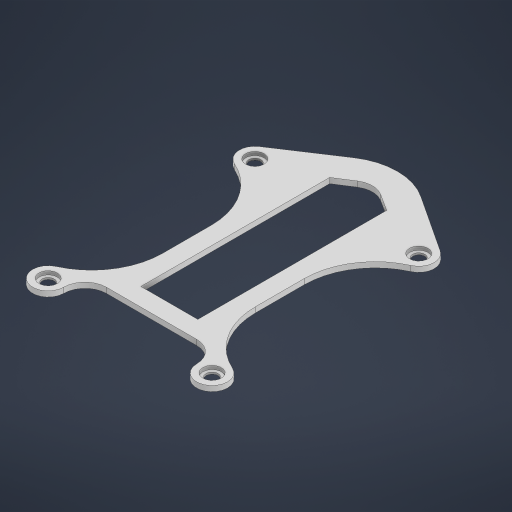
# Autodesk Inventor part: Skirt
Saved by Autodesk Inventor 2023 (Build 270158000, 158)
## iProperties
Created: 2022-10-14
Part Number: Skirt
Material: 一般
Document SubType Name: Modeling
Designer: hide
Density: 1 g/cm^3
Appearance: 既定
Author: hide
Autodesk Inventor part; units mm, degrees
ref_plane "YZ Plane" through (0, 0, 0) normal (1, 0, 0) x (0, 1, 0)
ref_plane "XZ Plane" through (0, 0, 0) normal (0, 1, 0) x (-1, 0, 0)
ref_plane "XY Plane" through (0, 0, 0) normal (0, 0, 1) x (1, 0, 0)
sketch "スケッチ1" plane through (0, 0, 0) normal (0, 1, 0) x (-1, 0, 0)
  circle A0 centre (11.5, 0) radius 0.85
  circle A1 centre (11.5, 29) radius 0.85
  line L0 (0, -11.6446) -> (0, 36.0381)
  arc A2 (12.3932, 27.0169) -> (9.325, 29) centre (11.5, 29) ccw
  arc A3 (12.6962, -1.8165) -> (12.3932, 1.9831) centre (11.5, 0) ccw
  circle A4 centre (0, 0) radius 5
  line L1 (4, 23.5) -> (4, -3)
  line L2 (4, -3) -> (1.6185, -4.5259)
  line L3 (12.6962, -1.8165) -> (4.675, -7.0989)
  arc A5 (0, -8.5) -> (4.675, -7.0989) centre (0, 0) ccw
  circle A6 centre (0, -2) radius 3
  line L4 (4, 23.5) -> (0, 23.5)
  line L5 (14.3325, 28.15) -> (9.1092, 28.15)
  line L6 (-4, 23.5) -> (-4, -3)
  line L7 (-4, -3) -> (-1.6185, -4.5259)
  line L8 (-4, 23.5) -> (0, 23.5)
  line L9 (6.5, 11.1009) -> (6.5, 17.8991)
  arc A7 (6.325, 26) -> (9.325, 29) centre (6.325, 29) ccw
  line L10 (6.325, 26) -> (0, 26)
  arc A8 (12.3932, 27.0169) -> (6.5, 17.8991) centre (16.5, 17.8991) ccw
  arc A9 (6.5, 11.1009) -> (12.3932, 1.9831) centre (16.5, 11.1009) ccw
  circle A10 centre (11.5, 0) radius 1.175
  circle A11 centre (11.5, 29) radius 1.175
  point P0 (0, 30.9357)
  point P1 (4, 3)
  point P2 (0, 26.5)
  point P3 (0, -5)
  point P4 (-1.6185, -4.5259)
  point P5 (0, 1)
  point P6 (-4, 3)
  point P7 (0, -5)
  point P8 (3.4728, -6.6475)
  point P9 (0, 5)
  point P10 (0, -5)
  point P11 (2.7322, -4.1875)
  point P12 (-4, -3)
  dimension "d7" = 10
  dimension "d2" = 29
  dimension "d18" = 8.5
  dimension "d24" = 1.7
  dimension "d25" = 2
  dimension "d39" = 8
  dimension "d41" = 2.5
  dimension "d43" = 2.5
  dimension "d44" = 10
  dimension "d45" = 23
  dimension "d47" = 3
  dimension "d48" = 2.35
  dimension "d49" = 1
  dimension "d50" = 1
  constraints: 20 end point, 12 point on circle, 10 centre point, 9 tangent, 6 coincident, 5 horizontal alignment, 3 equal radius, 2 horizontal, 1 vertical, 1 vertical alignment, 17 other
  measures "d2" distance of A1.centre A0.centre
  measures "d18" radius of A5
  measures "d24" diameter of A0
  measures "d25" distance of point (0, 0) point (0, -2)
  measures "d41" distance between parallel lines of L10 L4
  measures "d43" distance between parallel lines of L9 L1
  measures "d44" radius of A9
  measures "d47" radius of A7
  measures "d48" diameter of A10
  measures "d49" radial gap between concentric circles of A2 A11
  measures "d50" radial gap between concentric circles of A3 A10
extrude "押し出し1" add sketch "スケッチ1" along normal blind 0.75 contours L5 A11 | L5 A11 | A11 L5 A7 A2 | L5 A2 A8 L9 A9 A3 L3 A5 L0 A4 L1 L4 L10 A7 A11 | A4 L1 | A6 L2 A4 | A10
sketch "スケッチ2" plane through (0, 0.75, 0) normal (0, 1, 0) x (1, 0, 0)
  circle A0 centre (-11.5, 0) radius 1.3
  circle A1 centre (-11.5, 0) radius 0.85 projected
  circle A2 centre (-11.5, -29) radius 0.85 projected
  circle A3 centre (-11.5, -29) radius 0.85 projected
  circle A4 centre (-11.5, -29) radius 1.3
  point P0 (0, 0)
  dimension "d51" = 2.6
  constraints: 2 centre point, 2 coincident, 1 equal radius
  measures "d51" diameter of A0
extrude "押し出し2" cut sketch "スケッチ2" against normal blind 0.5
mirror "ミラー2" about plane through (0, 0, 26) normal (1, 0, 0) of "押し出し1", "押し出し2"
